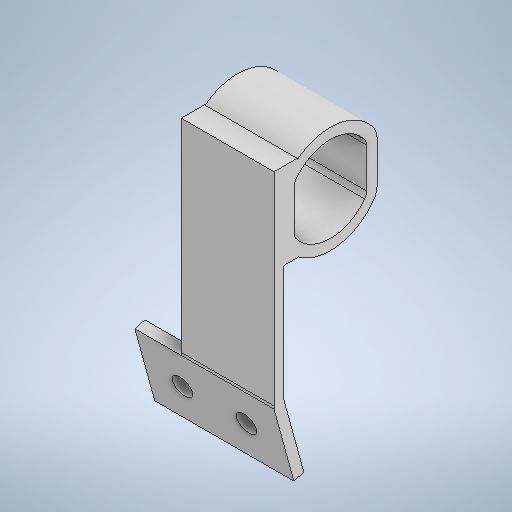
# Autodesk Inventor part: leftWheeler
Saved by Autodesk Inventor 2025.1 (Build 291241000, 241)
## iProperties
Created: 2025-06-15
Part Number: leftWheeler
Material: Generic
Document SubType Name: Modeling
Designer: User
Density: 1 g/cm^3
Appearance: Default
Author: User
## iProperties of the stored document rightWheeler_3DPrint.ipt
Created: 2025-06-15
Part Number: rightWheeler_3DPrint
Material: Generic
Document SubType Name: Modeling
Designer: User
Density: 1 g/cm^3
Appearance: Default
Author: User
Autodesk Inventor part; units mm, degrees
ref_plane "YZ Plane" through (0, 0, 0) normal (1, 0, 0) x (0, 1, 0)
ref_plane "XZ Plane" through (0, 0, 0) normal (0, 1, 0) x (-1, 0, 0)
ref_plane "XY Plane" through (0, 0, 0) normal (0, 0, 1) x (1, 0, 0)
sketch "Sketch1" plane through (0, 0, 0) normal (0, 0, 1) x (1, 0, 0)
  line L0 (1, 9) -> (14, 9) projected
  line L1 (1, 3) -> (1, 9) projected
  line L2 (14, 3) -> (1, 3) projected
  line L3 (14, 9) -> (14, 3) projected
  line L4 (1, 12) -> (14, 12)
  line L5 (1, 0) -> (14, 0)
  line L6 (1, 12.5) -> (14, 12.5)
  line L7 (1, -0.5) -> (14, -0.5)
  line L8 (0, 1.4) -> (0, 10.6) projected
  line L9 (0, -0.5) -> (14, -0.5)
  line L10 (14, -0.5) -> (14, 12.5)
  line L11 (14, 12.5) -> (0, 12.5)
  line L12 (0, 12.5) -> (0, -0.5)
  point P0 (0, 0)
  dimension "d0" = 0.5
  dimension "d1" = 0.5
  constraints: 16 end point, 4 parallel, 3 horizontal, 1 perpendicular, 4 other
  measures "d0" distance between parallel lines of L4 L6
  measures "d1" distance between parallel lines of L5 L7
extrude "Extrusion1" add sketch "Sketch1" along normal blind 2
sketch "Sketch2" plane through (14, -0.5, 0) normal (1, 0, 0) x (0, 0, -1)
  line L0 (10, 9.5) -> (10, 3.5) projected
  line L1 (10.5, 9.5) -> (10.5, 3.5)
  line L2 (0, 13) -> (0, 0) projected
  line L3 (0.0028, 13) -> (0, 0)
  arc A0 (5, 0.5) -> (9.8, 2.9) centre (5, 6.5) ccw projected
  spline S0 degree 3 poles (9.8, 10.1) (9.3822, 10.6561) (8.439, 11.5426) (6.738, 12.3306) (5.0002, 12.5848) (3.2616, 12.3308) (1.5615, 11.5422) (0.6175, 10.6564) (0.2, 10.1) knots 0.000048 0.000048 0.000048 0.000048 1.982593 3.634064 5.285536 6.937008 8.58848 10.571071 10.571071 10.571071 10.571071 weights 1 1 1 1 1 1 1 1 1 projected
  arc A1 (0.2, 2.9) -> (5, 0.5) centre (5, 6.5) ccw projected
  ellipse E0 centre (0.7683, 3.4229) end of major axis (0.4925, 4.2518) minor radius 0.7558 (0, 3.5) -> (0.2, 2.9) ccw projected
  ellipse E1 centre (0.7685, 9.5775) end of major axis (1.0457, 10.4061) minor radius 0.7558 (0.2, 10.1) -> (0, 9.5) ccw projected
  ellipse E2 centre (9.2317, 3.4229) end of major axis (9.5075, 4.2518) minor radius 0.7558 (9.8, 2.9) -> (10, 3.5) ccw projected
  ellipse E3 centre (9.2318, 9.5768) end of major axis (8.9568, 10.4058) minor radius 0.7558 (10, 9.5) -> (9.7999, 10.1) ccw projected
  arc A2 (5, 0.0295) -> (10.1758, 2.6168) centre (5, 6.5) ccw
  arc A3 (-0.1717, 2.6115) -> (5, 0.0295) centre (5, 6.5) ccw
  line L4 (10.4705, 3.4977) -> (10.4705, 9.5023)
  ellipse E4 centre (0.7683, 3.4229) end of major axis (0.3339, 4.718) minor radius 1.2242 (-0.4709, 3.5051) -> (-0.1717, 2.6115) ccw
  ellipse E5 centre (0.7685, 9.5775) end of major axis (1.1957, 10.8767) minor radius 1.2233 (-0.1748, 10.3845) -> (-0.4697, 9.4882) ccw
  arc A4 (0.2, 2.9) -> (9.8, 2.9) centre (5, 6.5) ccw projected
  arc A5 (5, -1.5631) -> (11.4481, 1.6589) centre (5, 6.5) ccw
  arc A6 (-1.4235, 1.6263) -> (5, -1.5631) centre (5, 6.5) ccw
  line L5 (12.0631, 3.4977) -> (12.0631, 9.5023)
  ellipse E6 centre (0.7683, 3.4229) end of major axis (-0.2657, 6.5587) minor radius 2.7801 (-2.0629, 3.5774) -> (-1.4235, 1.6263) ccw
  ellipse E7 centre (0.7685, 9.5775) end of major axis (1.7896, 12.7173) minor radius 2.7798 (-1.4322, 11.3622) -> (-2.0617, 9.4138) ccw
  line L6 (-0.4709, 3.5051) -> (-0.4697, 9.4882)
  line L7 (-2.0629, 3.5774) -> (-2.0617, 9.4138)
  spline S1 degree 5 poles (10.1762, 10.3826) (9.455, 11.3411) (8.5153, 12.1382) (7.3995, 12.6912) (5.0003, 13.2497) (2.6, 12.6917) (1.4857, 12.137) (0.5444, 11.3415) (-0.1764, 10.3824) knots 0 0 0 0 0 0 0.499984 0.499984 0.499984 1 1 1 1 1 1
  spline S2 degree 3 poles (10.1759, 2.6167) (10.3655, 2.8683) (10.4707, 3.1827) (10.4707, 3.4977) knots 0 0 0 0 1 1 1 1
  spline S3 degree 3 poles (10.4707, 9.5023) (10.4707, 9.8173) (10.3655, 10.1318) (10.1757, 10.3833) knots 0 0 0 0 1 1 1 1
  spline S4 degree 4 poles (11.4481, 1.6589) (11.7448, 2.0529) (11.9559, 2.5113) (12.0631, 3.0045) (12.0631, 3.4977) knots 0 0 0 0 0 1 1 1 1 1
  spline S5 degree 4 poles (12.0631, 9.5023) (12.0631, 9.995) (11.9561, 10.4877) (11.7455, 10.9457) (11.4492, 11.3395) knots 0 0 0 0 0 1 1 1 1 1
  spline S6 degree 5 poles (11.4495, 11.3391) (10.5511, 12.5335) (9.3795, 13.5256) (7.9898, 14.2154) (5.0062, 14.9093) (2.0215, 14.2187) (0.6377, 13.5325) (-0.5334, 12.5493) (-1.4322, 11.3622) knots 0 0 0 0 0 0 0.500955 0.500955 0.500955 1 1 1 1 1 1
  point P0 (0, 0.5)
  point P1 (0, 10.6069)
  point P2 (0, 12.8255)
  point P3 (0, 0.1744)
  point P4 (0, 2.393)
  point P5 (0.0005, 2.3924)
  point P6 (0, 0.1743)
  point P7 (0.0027, 12.8276)
  point P8 (0.0023, 10.6096)
  constraints: 12 end point, 8 point on circle, 7 parallel, 4 centre point, 41 other
extrude "Extrusion2" add sketch "Sketch2" along normal blind 2 contours L3 S6 S5 L5 S4 A5 A6 L2 A3 A2 S2 L4 S3 S1 | S1 E5 L6 E4 A3 L2 A6 E6 L7 E7 S6
sketch "Sketch3" plane through (14, 1.893, 0) normal (1, 0, 0) x (0, 0, -1)
  arc A0 (-0.1717, 0.2185) -> (0, 0) centre (5, 4.107) ccw projected
  line L0 (0, 0) -> (0, 8.2139) projected
  arc A1 (0, 8.2139) -> (-0.1748, 7.9915) centre (4.9785, 4.1209) ccw projected
  ellipse E0 centre (0.7685, 7.1845) end of major axis (0.3413, 5.8853) minor radius 1.2233 (-0.1748, 7.9915) -> (-0.4697, 7.0952) ccw projected
  line L1 (-0.4697, 7.0952) -> (-0.4709, 1.1121) projected
  ellipse E1 centre (0.7683, 1.03) end of major axis (1.2028, -0.2651) minor radius 1.2242 (-0.4709, 1.1121) -> (-0.1717, 0.2185) ccw projected
  point P0 (0, -1.893)
  constraints: 2 other
extrude "Extrusion3" cut sketch "Sketch3" against normal through all
sketch "Sketch4" plane through (14, -0.5, 0) normal (-1, 0, 0) x (0, 0, 1)
  line L0 (-10.4705, 9.5023) -> (-10.4705, 3.4977) projected
  ellipse E0 centre (-9.2512, 9.5832) end of major axis (-8.8307, 10.8511) minor radius 1.2058 (-10.1756, 10.3833) -> (-10.4705, 9.5023) ccw projected
  spline S0 degree 5 poles (-0.0023, 10.6096) (-0.7281, 11.4914) (-1.6474, 12.2152) (-2.7157, 12.7179) (-5.0579, 13.2362) (-7.3991, 12.6912) (-8.5148, 12.1385) (-9.4545, 11.3415) (-10.1756, 10.3833) knots 0 0 0 0 0 0 0.487709 0.487709 0.487709 1 1 1 1 1 1 projected
  line L1 (-0.0027, 12.8276) -> (-0.0023, 10.6096) projected
  spline S1 degree 5 poles (-11.4492, 11.3395) (-10.5511, 12.5335) (-9.3795, 13.5256) (-7.9898, 14.2154) (-5.4174, 14.8137) (-2.8441, 14.3827) (-1.8061, 14.0228) (-0.8486, 13.496) (-0.0027, 12.8277) knots 0 0 0 0 0 0 0.581033 0.581033 0.581033 1 1 1 1 1 1 projected
  ellipse E1 centre (-9.2769, 9.5918) end of major axis (-8.3583, 12.3614) minor radius 2.7713 (-11.4492, 11.3395) -> (-12.0631, 9.5023) ccw projected
  line L2 (-12.0631, 3.4977) -> (-12.0631, 9.5023) projected
  ellipse E2 centre (-9.2769, 3.4079) end of major axis (-10.1984, 6.1767) minor radius 2.7712 (-12.0631, 3.4977) -> (-11.4481, 1.6589) ccw projected
  arc A0 (-11.4481, 1.6589) -> (0, 0.1743) centre (-5, 6.5) ccw projected
  line L3 (-0.0005, 2.3924) -> (0, 0.1743) projected
  arc A1 (-10.1758, 2.6168) -> (-0.0005, 2.3924) centre (-5, 6.5) ccw projected
  ellipse E3 centre (-9.2512, 3.4164) end of major axis (-9.673, 4.684) minor radius 1.2058 (-10.4705, 3.4977) -> (-10.1758, 2.6168) ccw projected
  point P0 (0, 0.5)
  constraints: 6 other
extrude "Extrusion4" add sketch "Sketch4" along normal up to surface (14 mm away)
sketch "Sketch6" plane through (16, -0.5, 0) normal (1, 0, 0) x (0, 0, -1)
  arc A0 (0.0005, 2.3924) -> (10.1758, 2.6168) centre (5, 6.5) ccw projected
  spline S0 degree 5 poles (0.0023, 10.6096) (0.7281, 11.4914) (1.6474, 12.2152) (2.7157, 12.7179) (5.0579, 13.2362) (7.3991, 12.6912) (8.5148, 12.1385) (9.4545, 11.3415) (10.1756, 10.3833) knots 0 0 0 0 0 0 0.487709 0.487709 0.487709 1 1 1 1 1 1 projected
  spline S1 degree 5 poles (11.4492, 11.3395) (10.5511, 12.5335) (9.3795, 13.5256) (7.9898, 14.2154) (5.4174, 14.8137) (2.8441, 14.3827) (1.8061, 14.0228) (0.8486, 13.496) (0.0027, 12.8277) knots 0 0 0 0 0 0 0.581033 0.581033 0.581033 1 1 1 1 1 1 projected
  arc A1 (0, 0.1743) -> (11.4481, 1.6589) centre (5, 6.5) ccw projected
  arc A2 (-1.4235, 1.6263) -> (0, 0.1744) centre (5, 6.5) ccw projected
  arc A3 (-0.1717, 2.6115) -> (0, 2.393) centre (5, 6.5) ccw projected
  ellipse E0 centre (0.7683, 3.4229) end of major axis (1.2028, 2.1279) minor radius 1.2242 (-0.4709, 3.5051) -> (-0.1717, 2.6115) ccw projected
  line L0 (0.0005, 2.3924) -> (0, 2.393)
  line L1 (0, 2.393) -> (0, 0) projected
  line L2 (0, 0.1743) -> (0, 0.1744)
  arc A4 (0, 10.6069) -> (-0.1748, 10.3845) centre (4.9785, 6.5139) ccw projected
  line L3 (0.0023, 10.6096) -> (0, 10.6069)
  ellipse E1 centre (3.3491, 8.1967) end of major axis (-1.5218, 3.4578) minor radius 5.6955 (0, 12.8255) -> (-1.4322, 11.3622) ccw projected
  line L4 (0.0027, 12.8276) -> (0.0023, 10.6096) projected
  line L5 (0, 12.8255) -> (0.0027, 12.8276)
  line L6 (-0.1748, 10.3845) -> (-1.4322, 11.3622)
  ellipse E2 centre (0.7685, 9.5775) end of major axis (1.7896, 12.7173) minor radius 2.7798 (-1.4322, 11.3622) -> (-2.0617, 9.4138) ccw projected
  ellipse E3 centre (0.7683, 3.4229) end of major axis (1.2028, 2.1279) minor radius 1.2242 (-0.4709, 3.5051) -> (-0.1717, 2.6115) ccw projected
  line L7 (-0.1717, 2.6115) -> (-1.4235, 1.6263)
  line L8 (0.8417, -0.4081) -> (0.8417, 1.5426)
  line L9 (0.8417, 11.4571) -> (0.8417, 13.4082)
  point P0 (0, 0.5)
  constraints: 16 end point, 2 point on circle, 2 point on line, 1 tangent, 1 vertical, 10 other
extrude "Extrusion5" add sketch "Sketch6" against normal up to surface (16 mm away)
sketch "Sketch7" plane through (0, 0, 2) normal (0, 0, 1) x (1, 0, 0)
  line L0 (14, 12.5) -> (0, 12.5) projected
  line L1 (0, 12.5) -> (0, -0.5) projected
  line L2 (0, -0.5) -> (14, -0.5) projected
  line L3 (14, -0.5) -> (14, 2.5472) projected
  line L4 (14, 2.5472) -> (14, 9.4474) projected
  line L5 (14, 9.4474) -> (14, 12.5) projected
  line L6 (-39.2246, -25.2311) -> (17.3435, -25.0166)
  line L7 (4.645, -14.0646) -> (-40.8761, -14.2372)
  line L8 (0, 12.5) -> (14, 12.5)
  line L9 (14, 12.5) -> (14, -25.0293)
  line L10 (14, -25.0293) -> (0, -25.0293)
  line L11 (0, -25.0293) -> (0, 12.5)
  line L12 (-49.2943, 75.5434) -> (-86.9993, 74.8219)
  line L13 (-86.9197, 53.822) -> (-75.9204, 54.0325)
  line L14 (14, -25.0293) -> (-7, -25.0293)
  line L15 (-7, -25.0293) -> (-7, -14.1088)
  line L16 (-7, -14.1088) -> (14, -14.1088)
  line L17 (14, -14.1088) -> (14, -25.0293)
  point P0 (0, 0)
  point P1 (0, -14.1088)
  dimension "d24" = 21
  constraints: 24 end point, 4 parallel, 2 horizontal, 2 perpendicular, 2 point on line, 12 other
  measures "d24" distance of L15.end L16.end
extrude "Extrusion6" add sketch "Sketch7" along normal blind 1.5 contours L5 L4 L3 L2 L1 L0 | L2 L9 L16 L11 | L9 L10 L11 L16 | L16 L11 L14 L15
sketch "Sketch8" plane through (0, 0, 3.5) normal (0, 0, 1) x (1, 0, 0)
  line L0 (-7, -14.1088) -> (-7, -25.0293) projected
  line L1 (14, -25.0293) -> (14, 12.5) projected
  line L2 (14, -19.569) -> (9, -19.569)
  line L3 (-7, -19.569) -> (-2, -19.569)
  circle A0 centre (-2, -19.569) radius 1.5
  circle A1 centre (9, -19.569) radius 1.5
  point P0 (0, 0)
  dimension "d27" = 5
  dimension "d28" = 5
  dimension "d29" = 3
  dimension "d30" = 3
  constraints: 4 end point, 2 centre point, 2 coincident, 1 midpoint, 1 point on line
  measures "d27" distance of L2.start L2.end
  measures "d28" distance of L3.start L3.end
  measures "d29" diameter of A0
  measures "d30" diameter of A1
extrude "Extrusion7" cut sketch "Sketch8" against normal blind 1.5
sketch "Sketch9" plane through (0, 0, 3.5) normal (0, 0, 1) x (1, 0, 0)
  line L0 (16, 10.8395) -> (16, 14.0632) projected
  line L1 (16, 8.9138) -> (16, 10.8622) projected
  line L2 (16, 8.9138) -> (16, 3.0774) projected
  line L3 (16, 1.1263) -> (16, 3.0774) projected
  line L4 (16, -2.0631) -> (16, 1.1589) projected
  line L5 (14, -25.0293) -> (14, 12.5) projected
  line L6 (16, 14.0632) -> (14, 14.0632)
  line L7 (14, 14.0632) -> (14, -2.0631)
  line L8 (14, -2.0631) -> (16, -2.0631)
  line L9 (16, -2.0631) -> (16, 14.0632)
  point P0 (0, 0)
  point P1 (16, 12.3276)
  point P2 (14, 12.5)
  constraints: 8 end point, 2 parallel, 1 horizontal, 1 perpendicular, 1 point on line
extrude "Extrusion8" cut sketch "Sketch9" against normal blind 19
sketch "Sketch10" plane through (14, 2.9977, -12.0631) normal (1, 0, 0) x (0, 0, -1)
  line L0 (-14.0631, -17.1065) -> (-15.5631, -17.1065) projected
  line L1 (-15.5631, -28.027) -> (-15.5631, 9.5023) projected
  line L2 (-14.0631, -28.027) -> (-14.0631, -3.4977) projected
  line L3 (-11.0631, -28.027) -> (-14.0631, -17.1065)
  line L4 (-11.0631, -28.027) -> (-12.5095, -28.4243)
  line L5 (-12.5095, -28.4243) -> (-15.5631, -17.1065)
  point P0 (-12.0631, -2.9977)
  dimension "d36" = 1.5
  dimension "d49" = 11.325
  dimension "d50" = 11.3178
  constraints: 6 end point, 1 perpendicular
  measures "d36" distance of L3.start L4.end
  measures "d49" distance of L3.start L0.start
  measures "d50" vertical distance of L4.end L0.end
extrude "Extrusion9" add sketch "Sketch10" against normal up to surface (21 mm away)
sketch "Sketch11" plane through (14, 2.9977, -12.0631) normal (1, 0, 0) x (0, 0, -1)
  line L0 (-15.5631, -28.027) -> (-15.5631, 9.5023) projected
  line L1 (-14.0631, -28.027) -> (-14.0631, -22.6661) projected
  line L2 (-14.0631, -28.027) -> (-15.5631, -28.027) projected
  line L3 (-14.0631, -17.1065) -> (-15.5631, -17.1065) projected
  line L4 (-14.0631, -22.6661) -> (-12.5095, -28.4243) construction
  line L5 (-12.5095, -28.4243) -> (-15.5631, -17.1065)
  point P0 (-12.0631, -2.9977)
  point P1 (-14.0631, -22.6661)
  constraints: 2 end point
extrude "Extrusion10" cut sketch "Sketch11" against normal through all
sketch "Sketch12" plane through (-7, -25.4266, 0.4464) normal (0, -0.2604892, 0.9654768) x (1, 0, 0)
  line L0 (0, 0) -> (0, 11.7225) projected
  line L1 (21, 0) -> (0, 0) projected
  line L2 (21, 11.7225) -> (21, 0) projected
  line L3 (7, 11.7225) -> (21, 11.7225) projected
  line L4 (7, 11.7225) -> (0, 11.7225) projected
  line L5 (21, 11.3318) -> (7, 11.3318) projected
  line L6 (7, 11.3318) -> (0, 11.3318) projected
  circle A0 centre (5.6659, 5.6659) radius 5.6659
  circle A1 centre (15.3341, 5.6659) radius 5.6659
  circle A2 centre (5.6659, 5.6659) radius 1.5
  circle A3 centre (15.3341, 5.6659) radius 1.5
  point P0 (7, 24.4325)
  dimension "d41" = 3
  dimension "d42" = 3
  dimension "d51" = 11.3318
  constraints: 6 tangent, 4 centre point, 2 coincident
  measures "d41" diameter of A2
  measures "d42" diameter of A3
  measures "d51" diameter of A1
extrude "Extrusion11" cut sketch "Sketch12" against normal blind 10 contours A2 | A3
sketch "Sketch13" plane through (14, 2.9977, -12.0631) normal (1, 0, 0) x (0, 0, -1)
  line L0 (-15.5631, -17.1065) -> (-12.5095, -28.4243) projected
  line L1 (-11.0631, -28.027) -> (-14.0631, -17.1065) projected
  line L2 (-12.5095, -28.4243) -> (-11.0631, -28.027) projected
  line L3 (-15.5631, -17.1065) -> (-15.5631, 9.5023) projected
  line L4 (-14.0631, -17.1065) -> (-15.5631, -17.1065)
  point P0 (-12.0631, -2.9977)
  constraints: 2 end point, 1 perpendicular
extrude "Extrusion12" cut sketch "Sketch13" against normal through all
sketch "Sketch14" plane through (14, -14.1088, 2) normal (0, -1, 0) x (1, 0, 0)
  line L0 (-14, 0) -> (-14, 1.5) projected
  line L1 (0, 0) -> (-14, 0) projected
  line L2 (0, 1.5) -> (0, 0) projected
  line L3 (-14, 1.5) -> (0, 1.5) projected
  point P0 (-14, -2)
extrude "Extrusion13" add sketch "Sketch14" along normal blind 4
sketch "Sketch15" plane through (14, 2.9977, -12.0631) normal (1, 0, 0) x (0, 0, -1)
  line L0 (-14.0631, -21.1065) -> (-15.5631, -21.1065) projected
  line L1 (-14.0631, -21.1065) -> (-11.0631, -21.1065)
  line L2 (-14.0631, -3.4977) -> (-14.0631, -21.1065) projected
  line L3 (-14.0631, -21.1065) -> (-11.0631, -32.0218)
  line L4 (-15.5631, 9.5023) -> (-15.5631, -21.1065) projected
  line L5 (-15.5631, -21.1065) -> (-15.5631, -21.5188)
  line L6 (-15.5631, -21.5188) -> (-12.5631, -32.434)
  line L7 (-12.5631, -32.434) -> (-11.0631, -32.0218)
  point P0 (-12.0631, -2.9977)
  dimension "d52" = 3
  dimension "d53" = 11.32
  constraints: 10 end point, 1 horizontal, 1 perpendicular, 1 vertical
  measures "d52" distance of L0.start L1.end
  measures "d53" distance of L0.start L3.end
extrude "Extrusion14" add sketch "Sketch15" against normal up to surface (14 mm away)
sketch "Sketch16" plane through (0, 2.9977, -12.0631) normal (-1, 0, 0) x (0, 0, 1)
  line L0 (15.5631, -21.5188) -> (12.5631, -32.434) projected
  line L1 (11.0631, -32.0218) -> (14.0631, -21.1065) projected
  line L2 (15.5631, -21.5188) -> (14.0631, -21.1065)
  line L3 (14.0631, -21.1065) -> (11.0631, -32.0218)
  line L4 (11.0631, -32.0218) -> (12.5631, -32.434)
  line L5 (12.5631, -32.434) -> (15.5631, -21.5188)
  point P0 (12.0631, -2.9977)
  point P1 (12.5631, -32.434)
  constraints: 8 end point, 2 parallel, 2 perpendicular
extrude "Extrusion15" add sketch "Sketch16" along normal blind 7
sketch "Sketch17" plane through (-7, -29.4363, 0.5) normal (0, -0.2650177, 0.9642436) x (1, 0, 0)
  line L0 (21, 0) -> (0, 0) projected
  line L1 (21, 11.32) -> (21, 0) projected
  line L2 (21, 11.32) -> (7, 11.32) projected
  line L3 (7, 11.32) -> (0, 11.32) projected
  line L4 (0, 0) -> (0, 11.32) projected
  circle A0 centre (5.66, 5.66) radius 5.66
  circle A1 centre (15.34, 5.66) radius 5.66
  circle A2 centre (15.34, 5.66) radius 1.5
  circle A3 centre (5.66, 5.66) radius 1.5
  point P0 (7, 28.2513)
  dimension "d58" = 3
  dimension "d59" = 3
  constraints: 6 tangent, 4 centre point, 2 coincident
  measures "d58" diameter of A2
  measures "d59" diameter of A3
extrude "Extrusion16" cut sketch "Sketch17" against normal through all contours A2 | A3
body "Solid1"
